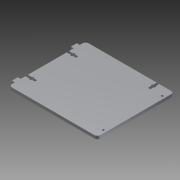
# Autodesk Inventor part: pieza protectora ramps
Saved by Autodesk Inventor 2012 (Build 160160000, 160)
## iProperties
Created: 2014-12-15
Part Number: pieza protectora ramps
Material: Default
Document SubType Name: Modeling
Designer: PRINCIPAL
Density: 1 g/cm^3
Author: PRINCIPAL
Autodesk Inventor part; units mm, degrees
ref_plane "YZ Plane" through (0, 0, 0) normal (1, 0, 0) x (0, 1, 0)
ref_plane "XZ Plane" through (0, 0, 0) normal (0, 1, 0) x (-1, 0, 0)
ref_plane "XY Plane" through (0, 0, 0) normal (0, 0, 1) x (1, 0, 0)
sketch "Boceto1" plane through (0, 0, 0) normal (0, 0, 1) x (1, 0, 0)
  line L0 (0, 0) -> (150, 0)
  line L1 (150, 0) -> (150, -130)
  line L2 (150, -130) -> (0, -130)
  line L3 (0, -130) -> (0, 0)
  dimension "d2" = 130
  dimension "d3" = 150
  constraints: 8 end point, 2 parallel, 1 horizontal, 1 perpendicular
  measures "d2" distance between parallel lines of L2 L0
  measures "d3" distance between parallel lines of L1 L3
extrude "Extrusión1" add sketch "Boceto1" along normal blind 5
fillet "Empalme1" radius 5 4 edges at (150, -130, 2.5) (150, 0, 2.5) (0, 0, 2.5) (0, -130, 2.5)
sketch "Boceto2" plane through (0, 0, 5) normal (0, 0, 1) x (1, 0, 0)
  line L0 (0, -125) -> (0, -5) projected
  line L1 (0, -10) -> (-5, -10)
  line L2 (-5, -10) -> (-5, -20)
  line L3 (-5, -20) -> (0, -20)
  line L4 (0, -20) -> (0, -10)
  line L5 (0, -110) -> (-5, -110)
  line L6 (-5, -110) -> (-5, -120)
  line L7 (-5, -120) -> (0, -120)
  line L8 (0, -120) -> (0, -110)
  line L9 (5, 0) -> (145, 0) projected
  point P0 (0, 0)
  dimension "d5" = 10
  dimension "d6" = 10
  dimension "d7" = 5
  dimension "d8" = 5
  dimension "d11" = 10
  dimension "d12" = 110
  constraints: 16 end point, 4 parallel, 2 horizontal, 2 perpendicular, 2 point on line
  measures "d5" distance between parallel lines of L3 L1
  measures "d6" distance between parallel lines of L7 L5
  measures "d7" distance between parallel lines of L8 L6
  measures "d8" distance between parallel lines of L4 L2
  measures "d11" distance from line of L1.end L9
  measures "d12" distance between parallel lines of L5 L9
extrude "Extrusión2" add sketch "Boceto2" against normal blind 5
sketch "Boceto3" plane through (0, 0, 5) normal (0, 0, 1) x (1, 0, 0)
  line L0 (-5, -20) -> (0, -20) projected
  line L1 (0, -110) -> (0, -20) projected
  line L2 (-0.1512, -97.9504) -> (7.0488, -97.9504)
  line L3 (7.0488, -97.9504) -> (7.0488, -96.7034)
  line L4 (7.0488, -96.7034) -> (10.0488, -96.7034)
  line L5 (10.0488, -96.7034) -> (10.0488, -97.9504)
  line L6 (10.0488, -97.9504) -> (15.7176, -97.9504)
  line L7 (15.7176, -97.9504) -> (15.7176, -102)
  line L8 (15.7176, -102) -> (10.0488, -102)
  line L9 (10.0488, -102) -> (10.0488, -103.247)
  line L10 (10.0488, -103.247) -> (7.0488, -103.247)
  line L11 (7.0488, -103.247) -> (7.0488, -102)
  line L12 (7.0488, -102) -> (-0.1512, -102)
  line L13 (10.0793, -33.2966) -> (7.0793, -33.2966)
  line L14 (7.0793, -33.2966) -> (7.0793, -32.0496)
  line L15 (10.0793, -32.0496) -> (10.0793, -33.2966)
  line L16 (7.0793, -32.0496) -> (-0.1207, -32.0496)
  line L17 (15.7481, -32.0496) -> (10.0793, -32.0496)
  line L18 (-0.1207, -28) -> (7.0793, -28)
  line L19 (15.7481, -28) -> (15.7481, -32.0496)
  line L20 (7.0793, -28) -> (7.0793, -26.753)
  line L21 (7.0793, -26.753) -> (10.0793, -26.753)
  line L22 (10.0793, -26.753) -> (10.0793, -28)
  line L23 (10.0793, -28) -> (15.7481, -28)
  line L24 (-0.1207, -28) -> (-0.1207, -32.0496)
  line L25 (-0.1512, -97.9504) -> (-0.1512, -102)
  point P0 (0, 0)
  dimension "d15" = 8
  dimension "d16" = 8
  constraints: 48 end point, 2 parallel
  measures "d15" distance from line of L12 L1.start
  measures "d16" distance between parallel lines of L18 L0
extrude "Extrusión3" cut sketch "Boceto3" against normal blind 10
sketch "Boceto4" plane through (0, 0, 5) normal (0, 0, 1) x (1, 0, 0)
  line L0 (125, 0.788) -> (125, -6.2913)
  line L1 (125, -6.2913) -> (126.247, -6.2913)
  line L2 (126.247, -6.2913) -> (126.247, -9.2913)
  line L3 (126.247, -9.2913) -> (125, -9.2913)
  line L4 (125, -9.2913) -> (125, -14.9601)
  line L5 (125, -14.9601) -> (120.9504, -14.9601)
  line L6 (120.9504, -14.9601) -> (120.9504, -9.2913)
  line L7 (120.9504, -9.2913) -> (119.7034, -9.2913)
  line L8 (119.7034, -9.2913) -> (119.7034, -6.2913)
  line L9 (119.7034, -6.2913) -> (120.9504, -6.2913)
  line L10 (120.9504, -6.2913) -> (120.9504, 0.788)
  line L11 (120.9504, 0.788) -> (125, 0.788)
  point P0 (0, 0)
  point P1 (150, -5)
  dimension "d22" = 25
  constraints: 24 end point, 1 perpendicular
  measures "d22" distance from line of point (150, -5) L0
extrude "Extrusión4" cut sketch "Boceto4" against normal blind 10
sketch "Boceto5" plane through (0, 0, 5) normal (0, 0, 1) x (1, 0, 0)
  circle A0 centre (145, -115) radius 1.75
  circle A1 centre (145, -15) radius 1.75
  point P0 (0, 0)
  dimension "d24" = 3.5
  dimension "d25" = 3.5
  constraints: 2 centre point
  measures "d24" diameter of A0
  measures "d25" diameter of A1
extrude "Extrusión5" cut sketch "Boceto5" against normal blind 10
